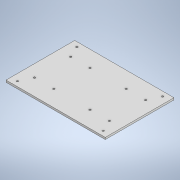
# Autodesk Inventor part: base
Saved by Autodesk Inventor 2022 (Build 260153000, 153)
## iProperties
Created: 2022-04-10
Part Number: base
Material: Generic
Document SubType Name: Modeling
Designer: Cody
Density: 1 g/cm^3
Appearance: Default
Author: Cody
Autodesk Inventor part; units mm, degrees
ref_plane "YZ Plane" through (0, 0, 0) normal (1, 0, 0) x (0, 1, 0)
ref_plane "XZ Plane" through (0, 0, 0) normal (0, 1, 0) x (-1, 0, 0)
ref_plane "XY Plane" through (0, 0, 0) normal (0, 0, 1) x (1, 0, 0)
sketch "Sketch1" plane through (0, 0, 0) normal (0, 1, 0) x (-1, 0, 0)
  line L0 (-162.5, 112.5) -> (162.5, 112.5)
  line L1 (162.5, 112.5) -> (162.5, -112.5)
  line L2 (162.5, -112.5) -> (-162.5, -112.5)
  line L3 (-162.5, -112.5) -> (-162.5, 112.5)
  line L4 (-162.5, 112.5) -> (162.5, -112.5) construction
  line L5 (162.5, 112.5) -> (-162.5, -112.5) construction
  line L6 (-140.3856, -97.19) -> (140.3856, -97.19) construction
  line L7 (140.3856, -97.19) -> (140.3856, 97.19) construction
  line L8 (140.3856, 97.19) -> (-140.3856, 97.19) construction
  line L9 (-140.3856, 97.19) -> (-140.3856, -97.19) construction
  line L10 (-140.3856, -97.19) -> (140.3856, 97.19) construction
  line L11 (140.3856, -97.19) -> (-140.3856, 97.19) construction
  circle A0 centre (140.3856, 97.19) radius 3
  line L12 (0, 467.949) -> (0, -391.4434) construction
  line L13 (289.9763, 0) -> (-240.0681, 0) construction
  circle A1 centre (140.3856, -97.19) radius 3
  circle A2 centre (-140.3856, 97.19) radius 3
  circle A3 centre (-140.3856, -97.19) radius 3
  point P0 (0, 0)
  dimension "d0" = 325
  dimension "d1" = 225
  dimension "d6" = 6
  constraints: 28 end point, 4 centre point, 4 midpoint, 4 parallel, 3 horizontal, 3 symmetric about line, 2 perpendicular, 2 point on line, 1 coincident, 1 vertical, 3 other
  measures "d0" distance of L1.end L2.end
  measures "d1" distance of L0.end L1.end
  measures "d6" diameter of A0
extrude "Extrusion1" add sketch "Sketch1" along normal blind 6.35
sketch "Sketch3" plane through (0, 6.35, 0) normal (0, 1, 0) x (1, 0, 0)
  line L0 (-122.75, -59.25) -> (122.75, -59.25) construction
  line L1 (122.75, -59.25) -> (122.75, 59.25) construction
  line L2 (122.75, 59.25) -> (-122.75, 59.25) construction
  line L3 (-122.75, 59.25) -> (-122.75, -59.25) construction
  line L4 (-122.75, -59.25) -> (122.75, 59.25) construction
  line L5 (122.75, -59.25) -> (-122.75, 59.25) construction
  line L6 (-59.25, -59.25) -> (59.25, -59.25) construction
  line L7 (59.25, -59.25) -> (59.25, 59.25) construction
  line L8 (59.25, 59.25) -> (-59.25, 59.25) construction
  line L9 (-59.25, 59.25) -> (-59.25, -59.25) construction
  line L10 (-59.25, -59.25) -> (59.25, 59.25) construction
  line L11 (59.25, -59.25) -> (-59.25, 59.25) construction
  circle A0 centre (-122.75, 59.25) radius 3
  circle A1 centre (-59.25, 59.25) radius 3
  line L12 (0, 196.1664) -> (0, -273.9197) construction
  line L13 (-414.1758, 0) -> (534.2765, 0) construction
  circle A2 centre (-122.75, -59.25) radius 3
  circle A3 centre (-59.25, -59.25) radius 3
  line L14 (0, -196.1664) -> (0, 273.9197) construction
  circle A4 centre (-122.75, -59.25) radius 3
  circle A5 centre (-59.25, -59.25) radius 3
  circle A6 centre (122.75, 59.25) radius 3
  circle A7 centre (59.25, 59.25) radius 3
  circle A8 centre (59.25, -59.25) radius 3
  circle A9 centre (122.75, -59.25) radius 3
  point P0 (0, 0)
  dimension "d17" = 245.5
  dimension "d18" = 118.5
  dimension "d19" = 118.5
  dimension "d20" = 6
  constraints: 30 end point, 10 centre point, 10 symmetric about line, 4 midpoint, 4 parallel, 3 horizontal, 2 coincident, 2 perpendicular, 1 point on line, 1 vertical, 8 other
  measures "d17" distance of L2.end L1.end
  measures "d18" distance of L0.end L1.end
  measures "d19" distance of L8.end L7.end
  measures "d20" diameter of A0
extrude "Extrusion3" cut sketch "Sketch3" against normal up to surface (6.35 mm away)
body "Solid1"
